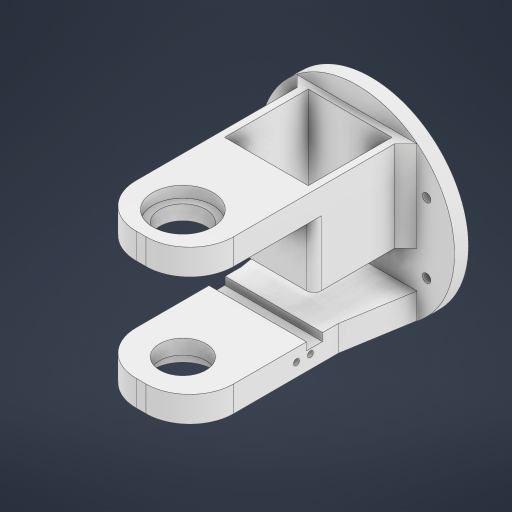
# Autodesk Inventor part: base
Saved by Autodesk Inventor 2024 (Build 280153000, 153)
## iProperties
Created: 2023-11-03
Part Number: base
Material: ABS Plastic
Document SubType Name: Modeling
Designer: mb
Density: 1.06 g/cm^3
Appearance: Smooth - White
Mass: 556.7 g
Surface Area: 852.672 cm^2
Volume: 525.188 cm^3
Author: mb
## iProperties of the stored document base_3DPrint.ipt
Created: 2024-02-22
Part Number: base_3DPrint
Material: Generic
Document SubType Name: Modeling
Designer: MaartenGeorgesBuelen
Density: 1 g/cm^3
Appearance: Default
Author: MaartenGeorgesBuelen
Autodesk Inventor part; units mm, degrees
ref_plane "YZ Plane" through (0, 0, 0) normal (1, 0, 0) x (0, 1, 0)
ref_plane "XZ Plane" through (0, 0, 0) normal (0, 1, 0) x (-1, 0, 0)
sketch "Sketch1" plane through (0, 0, 0) normal (0, 0, 1) x (1, 0, 0)
  circle A0 centre (0, 0) radius 70
  dimension "d0" = 140
  constraints: 1 centre point, 1 coincident
  measures "d0" diameter of A0
extrude "Extrusion1" add sketch "Sketch1" along normal blind 10
sketch "Sketch2" plane through (0, 0, 10) normal (0, 0, 1) x (1, 0, 0)
  line L0 (-35, -55) -> (35, -55)
  line L1 (35, -55) -> (35, -35)
  line L2 (35, -35) -> (-35, -35)
  line L3 (-35, -35) -> (-35, -55)
  line L4 (35, 35) -> (-35, 35)
  line L5 (-35, 35) -> (-35, 55)
  line L6 (-35, 55) -> (35, 55)
  line L7 (35, 55) -> (35, 35)
  circle A0 centre (0, 0) radius 70 projected
  line L8 (-35, -35) -> (-60.6218, -35)
  line L9 (35, 35) -> (60.6218, 35)
  line L10 (-35, 35) -> (-60.6218, 35)
  line L11 (35, -35) -> (60.6218, -35)
  dimension "d3" = 35
  dimension "d4" = 35
  dimension "d5" = 20
  dimension "d6" = 70
  dimension "d7" = 35
  constraints: 24 end point, 5 horizontal, 4 parallel, 4 point on circle, 2 equal length, 2 perpendicular, 2 point on line
  measures "d3" distance from line of point (0, 0) L2
  measures "d4" distance from line of point (0, 0) L4
  measures "d5" distance of L2.end L0.start
  measures "d6" distance of L0.start L0.end
  measures "d7" distance from line of point (0, 0) L3
extrude "Extrusion2" add sketch "Sketch2" along normal blind 155 contours L3 L2 L1 L0 | L5 L6 L7 L4
sketch "Sketch4" plane through (-35, 35, 10) normal (0, -1, 0) x (1, 0, 0)
  line L0 (70, 0) -> (70, 155) projected
  line L1 (0, 66) -> (70, 66)
  line L2 (70, 66) -> (70, 0)
  line L3 (70, 0) -> (0, 0)
  line L4 (0, 0) -> (0, 66)
  line L5 (0, 66) -> (70, 0) construction
  line L6 (70, 66) -> (0, 0) construction
  circle A0 centre (58.5, 11.5) radius 3 projected
  circle A1 centre (58.5, 58.5) radius 3 projected
  circle A2 centre (11.5, 11.5) radius 3 projected
  circle A3 centre (11.5, 58.5) radius 3 projected
  line L7 (62.5, 62.5) -> (7.5, 62.5) projected
  line L8 (7.5, 62.5) -> (7.5, 7.5) projected
  line L9 (7.5, 7.5) -> (62.5, 7.5) projected
  line L10 (62.5, 7.5) -> (62.5, 62.5) projected
  circle A4 centre (35, 35) radius 20 projected
  circle A5 centre (35, 35) radius 23
  point P0 (35, -10)
  dimension "d77" = 3
  constraints: 12 end point, 2 parallel, 1 centre point, 1 horizontal, 1 perpendicular
  measures "d77" radial gap between concentric circles of A4 A5
extrude "Extrusion4" add sketch "Sketch4" along normal blind 45 contours L3 L4 L1 L0 | L10 L9 L8 L7
sketch "Sketch3" plane through (-35, 55, 10) normal (0, 1, 0) x (1, 0, 0)
  line L0 (65, -65) -> (5, -65)
  line L1 (5, -65) -> (5, -5)
  line L2 (5, -5) -> (65, -5)
  line L3 (65, -5) -> (65, -65)
  line L4 (-35, 0) -> (105, 0) projected
  line L5 (70, 0) -> (70, -155) projected
  line L6 (35, 0) -> (35, -1.4267)
  point P0 (35, 10)
  dimension "d10" = 60
  dimension "d11" = 60
  dimension "d12" = 5
  constraints: 10 end point, 3 parallel, 1 horizontal, 1 midpoint, 1 perpendicular, 1 vertical, 1 other
  measures "d10" distance of L0.start L0.end
  measures "d11" distance of L2.end L0.start
  measures "d12" distance between parallel lines of L4 L2
extrude "Extrusion3" cut sketch "Sketch3" against normal blind 60
sketch "Sketch5" plane through (-35, 55, 165) normal (0, 1, 0) x (1, 0, 0)
  circle A0 centre (35, 30) radius 13.5
  line L0 (70, 155) -> (70, 0) projected
  line L1 (70, 0) -> (0, 0) projected
  circle A1 centre (35, 30) radius 16.5
  point P0 (35, 165)
  point P1 (70, 125)
  point P2 (70, 69)
  dimension "d28" = 35
  dimension "d29" = 30
  dimension "d40" = 27
  dimension "d84" = 3
  constraints: 2 centre point
  measures "d28" distance from line of L0 A0.centre
  measures "d29" distance from line of L1 A0.centre
  measures "d40" diameter of A0
  measures "d84" radial gap between concentric circles of A0 A1
extrude "Extrusion5" cut sketch "Sketch5" against normal through all contours A0 | A1
ref_plane "Work Plane2" through (-35, -55, 15) normal (0, -1, 0) x (1, 0, 0)
sketch "Sketch6" plane through (-35, -55, 15) normal (0, -1, 0) x (1, 0, 0)
  circle A0 centre (35, 120) radius 13.5
  circle A1 centre (35, 120) radius 21.5
  circle A2 centre (35, 120) radius 13.5 projected
  point P0 (35, -15)
  dimension "d35" = 8
  constraints: 2 centre point, 2 concentric
  measures "d35" radial gap between concentric circles of A0 A1
extrude "Extrusion6" cut sketch "Sketch6" against normal blind 8
ref_plane "Work Plane1" through (-40, 0, 10) normal (0, 1, 0) x (1, 0, 0)
offset faces "Size1" outward -1 faces at (0.663, -35, 46.2068) (-0.663, 35, 90.2068)
fillet "Fillet1" radius 31.5 4 edges at (-35, -45.5, 165) (35, -45.5, 165) (-35, 45.5, 165) (35, 45.5, 165)
sketch "Sketch7" plane through (0, 0, 10) normal (0, 0, 1) x (1, 0, 0)
  circle A0 centre (-50, 25) radius 3
  circle A1 centre (-50, -25) radius 3
  circle A2 centre (50, -25) radius 3
  circle A3 centre (50, 25) radius 3
  circle A4 centre (0, 15) radius 3
  circle A5 centre (0, -15) radius 3
  line L0 (-98, 0) -> (98, 0) projected
  line L1 (0, 0) -> (0, 59.6277)
  dimension "d41" = 25
  dimension "d42" = 25
  dimension "d43" = 50
  dimension "d44" = 50
  dimension "d45" = 15
  dimension "d46" = 15
  dimension "d47" = 25
  dimension "d48" = 25
  dimension "d49" = 50
  dimension "d50" = 50
  dimension "d51" = 6
  constraints: 6 centre point, 5 equal radius, 2 end point, 1 vertical
  measures "d41" distance from line of L0 A0.centre
  measures "d42" distance from line of L0 A1.centre
  measures "d43" distance from line of L1 A0.centre
  measures "d44" distance from line of L1 A1.centre
  measures "d45" distance from line of L0 A5.centre
  measures "d46" distance from line of L0 A4.centre
  measures "d47" distance from line of L0 A3.centre
  measures "d48" distance from line of L0 A2.centre
  measures "d49" distance from line of L1 A2.centre
  measures "d50" distance from line of L1 A3.centre
  measures "d51" diameter of A0
extrude "Extrusion7" cut sketch "Sketch7" against normal through all
fillet "Fillet2" radius 5.5 2 edges at (35, 13, 76) (-35, 13, 76)
ref_plane "Work Plane4" through (-35, -55, 15) normal (-1, 0, 0) x (0, 0, 1)
sketch "Sketch8" plane through (-35, -55, 15) normal (-1, 0, 0) x (0, 0, 1)
  line L0 (118.5, 19) -> (118.5, 0) projected
  line L1 (-5, 19) -> (118.5, 19) projected
  line L2 (-5, 0) -> (118.5, 0) projected
  circle A0 centre (73.5, 9.5) radius 2.1
  circle A1 centre (63.5, 9.5) radius 2.1
  line L3 (-5, 0) -> (-5, 19) projected
  point P0 (-15, 55)
  dimension "d55" = 10
  dimension "d56" = 4.2
  dimension "d57" = 9.5
  dimension "d58" = 45
  constraints: 2 centre point, 1 equal radius
  measures "d55" distance of A1.centre A0.centre
  measures "d56" diameter of A0
  measures "d57" distance from line of L2 A0.centre
  measures "d58" distance from line of L0 A0.centre
extrude "Extrusion8" cut sketch "Sketch8" against normal through all contours A0 | A1
chamfer "Chamfer4" distance 8 distance2 48.25 2 edges at (35, -45.5, 10) (-35, -45.5, 10) measured on face at (0.1205, -29.9927, 10)
chamfer "Chamfer5" distance 8 angle 45 2 edges at (35, 22.5, 10) (-35, 22.5, 10)
move faces "Move1" translate (0, 0.5, 0) faces at (0.663, 36, 90.2068)
move faces "Move2" translate (0, -0.5, 0) faces at (0.663, -36, 78.3734)
sketch "Sketch10" plane through (-3.5, 55, 165) normal (0, 1, 0) x (1, 0, 0)
  circle A0 centre (3.5, 30) radius 13.5 projected
  circle A1 centre (3.5, 30) radius 19
  circle A2 centre (3.5, 30) radius 21.5
  circle A3 centre (3.5, 30) radius 15.5
  point P0 (3.5, 165)
  dimension "d73" = 38
  dimension "d74" = 43
  dimension "d83" = 2
  constraints: 3 centre point, 2 coincident
  measures "d73" diameter of A1
  measures "d74" diameter of A2
  measures "d83" radial gap between concentric circles of A0 A3
extrude "Extrusion9" cut sketch "Sketch10" against normal blind 8 contours A0 | A1 | A2 | A3
sketch "Sketch11" plane through (-35, -55, 58.25) normal (-1, 0, 0) x (0, 0, 1)
  line L0 (0, 18.5) -> (75.25, 18.5) projected
  line L1 (12.25, 16) -> (12.25, 34.5) projected
  line L2 (22.25, 16) -> (12.25, 16) projected
  line L3 (22.25, 34.5) -> (22.25, 16) projected
  line L4 (12.25, 34.5) -> (22.25, 34.5) projected
  circle A0 centre (17.25, 25.5) radius 3.2 projected
  line L5 (22.25, 16) -> (12.25, 16)
  line L6 (12.25, 16) -> (12.25, 13)
  line L7 (12.25, 13) -> (22.25, 13)
  line L8 (22.25, 13) -> (22.25, 16)
  line L9 (22.25, 13) -> (23, 13)
  line L10 (23, 13) -> (23, 18.5)
  line L11 (23, 18.5) -> (22.25, 18.5)
  line L12 (22.25, 18.5) -> (22.25, 13)
  line L13 (12.25, 13) -> (11.5, 13)
  line L14 (11.5, 13) -> (11.5, 18.5)
  line L15 (11.5, 18.5) -> (12.25, 18.5)
  line L16 (12.25, 18.5) -> (12.25, 13)
  point P0 (-58.25, 55)
  dimension "d78" = 3
  dimension "d79" = 0.75
  dimension "d80" = 0.75
  constraints: 24 end point, 6 parallel, 3 horizontal, 3 perpendicular, 3 other
  measures "d78" distance of L6.end L5.end
  measures "d79" distance of L11.end L10.end
  measures "d80" distance of L14.end L15.end
extrude "Extrusion10" cut sketch "Sketch11" against normal through all contours L0 L1 L6 L13 L14 | L0 L3 L2 L1 | L0 L10 L9 L8 L3 | L2 L8 L7 L6
equation "\"d3\" = 0.5 * base_arm_widht"
equation "\"d4\" = 0.5 * base_arm_widht"
equation "\"base_arm_widht\" = 70"
body "Solid1"
